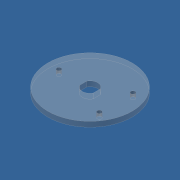
# Autodesk Inventor part: Couvercle_haut
Saved by Autodesk Inventor 2015 SP2 (Build 190223200, 223)
## iProperties
Created: 2018-03-26
Part Number: Couvercle_haut
Project: Nom Projet
Material: Plastique PMMA
Description: Nom pièce
Document SubType Name: Modeling
Designer: Alexandre.PICOTTE
Authority: brut Ø
Density: 1.188 g/cm^3
Appearance: Transparent - Clair
Author: Alexandre.PICOTTE
Material number: ---
Autodesk Inventor part; units mm, degrees
ref_plane "Plan YZ" through (0, 0, 0) normal (1, 0, 0) x (0, 1, 0)
ref_plane "Plan XZ" through (0, 0, 0) normal (0, 1, 0) x (-1, 0, 0)
ref_plane "Plan XY" through (0, 0, 0) normal (0, 0, 1) x (1, 0, 0)
sketch "Esquisse1" plane through (0, 0, 0) normal (0, 0, 1) x (1, 0, 0)
  circle A0 centre (0, 0) radius 25
  arc A1 (4, 2.1685) -> (-4, 2.1685) centre (0, 0) ccw
  line L0 (-4, -2.1685) -> (-4, 2.1685)
  arc A2 (-4, -2.1685) -> (4, -2.1685) centre (0, 0) ccw
  line L1 (4, -2.1685) -> (4, 2.1685)
  line L2 (0, -35) -> (0, 35) construction
  line L3 (-35, 0) -> (35, 0) construction
  point P0 (0, 0)
  dimension "d0" = 50
  dimension "d1" = 8
  dimension "d2" = 4.55
  constraints: 4 end point, 4 point on circle, 3 centre point, 2 parallel, 1 coincident, 1 vertical, 2 other
  measures "d0" diameter of A0
  measures "d1" distance between parallel lines of L1 L0
  measures "d2" radius of A2
extrude "Extrusion1" add sketch "Esquisse1" along normal blind 3
sketch "Esquisse6" plane through (0, 0, 3) normal (0, 0, 1) x (1, 0, 0)
  line L0 (-35, 0) -> (35, 0) construction
  line L1 (0, -35) -> (0, 35) construction
  circle A0 centre (0, 0) radius 18.5 construction
  point P0 (-18.5, 0)
  point P1 (15.5644, -10)
  point P2 (15.5644, 10)
  dimension "d5" = 37
  dimension "d6" = 20
  constraints: 3 point on circle, 1 centre point, 1 coincident, 1 point on line, 1 symmetric about line
  measures "d5" diameter of A0
  measures "d6" distance of point (15.564, 10) A0.end
hole "Perçage1" at (-18.5, 0, 3) at (15.5644, -10, 3) at (15.5644, 10, 3) direction (0, 0, -1) diameter 2.459 end through all thread size "M3x0.5" class "6H" standard "ISO M"
